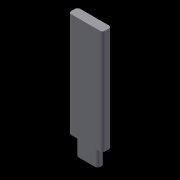
# Autodesk Inventor part: 3d_JacintoDevKit_Addon - USB Type-C
Saved by Autodesk Inventor 2018.3 (Build 223284000, 284)
## iProperties
Created: 2026-02-25
Part Number: 3d_JacintoDevKit_Addon - USB Type-C
Material: Genérico
Document SubType Name: Modeling
Designer: aca6
Density: 1 g/cm^3
Appearance: Valor por defecto
Author: aca6
Autodesk Inventor part; units mm, degrees
ref_plane "YZ Plane" through (0, 0, 0) normal (1, 0, 0) x (0, 1, 0)
ref_plane "XZ Plane" through (0, 0, 0) normal (0, 1, 0) x (-1, 0, 0)
ref_plane "XY Plane" through (0, 0, 0) normal (0, 0, 1) x (1, 0, 0)
sketch "Sketch1" plane through (0, 0, 0) normal (0, 0, 1) x (1, 0, 0)
  line L0 (-5.5, 1.75) -> (5.5, 1.75)
  line L1 (6.5, 0.75) -> (6.5, -0.75)
  line L2 (5.5, -1.75) -> (-5.5, -1.75)
  line L3 (-6.5, -0.75) -> (-6.5, 0.75)
  line L4 (0, 0) -> (0, 3.6789) construction
  line L5 (0, 0) -> (3.0794, 0) construction
  arc A0 (-5.5, 1.75) -> (-6.5, 0.75) centre (-5.5, 0.75) ccw
  arc A1 (-6.5, -0.75) -> (-5.5, -1.75) centre (-5.5, -0.75) ccw
  arc A2 (5.5, -1.75) -> (6.5, -0.75) centre (5.5, -0.75) ccw
  arc A3 (6.5, 0.75) -> (5.5, 1.75) centre (5.5, 0.75) ccw
  point P0 (-6.5, 1.75)
  point P1 (6.5, -1.75)
  point P2 (6.5, 1.75)
  dimension "d0" = 13
  dimension "d1" = 3.5
  dimension "d2" = 1
  dimension "d3" = 1
  constraints: 12 end point, 8 point on circle, 8 tangent, 6 point on line, 4 centre point, 3 horizontal, 2 equal radius, 2 parallel, 2 perpendicular, 1 vertical, 4 other
  measures "d0" distance of point (-6.5, 1.75) point (6.5, 1.75)
  measures "d1" distance of point (6.5, 1.75) point (6.5, -1.75)
  measures "d2" radius of A0
  measures "d3" radius of A1
extrude "Extrusion1" add sketch "Sketch1" along normal blind 40
sketch "Sketch2" plane through (0, 0, 0) normal (0, 0, -1) x (-1, 0, 0)
  line L0 (-3.15, 1.25) -> (3.15, 1.25)
  line L1 (4.15, 0.25) -> (4.15, -0.25)
  line L2 (3.15, -1.25) -> (-3.15, -1.25)
  line L3 (-4.15, -0.25) -> (-4.15, 0.25)
  line L4 (0, 0) -> (0, 2.3167) construction
  line L5 (0, 0) -> (2.0938, 0) construction
  arc A0 (-3.15, 1.25) -> (-4.15, 0.25) centre (-3.15, 0.25) ccw
  arc A1 (-4.15, -0.25) -> (-3.15, -1.25) centre (-3.15, -0.25) ccw
  arc A2 (3.15, -1.25) -> (4.15, -0.25) centre (3.15, -0.25) ccw
  arc A3 (4.15, 0.25) -> (3.15, 1.25) centre (3.15, 0.25) ccw
  point P0 (4.15, -1.25)
  point P1 (4.15, 1.25)
  point P2 (-4.15, -1.25)
  dimension "d6" = 8.3
  dimension "d7" = 2.5
  dimension "d8" = 1
  constraints: 12 end point, 8 point on circle, 8 tangent, 6 point on line, 4 centre point, 3 equal radius, 3 horizontal, 2 parallel, 2 vertical, 1 perpendicular, 4 other
  measures "d6" distance of point (4.15, -1.25) point (-4.15, -1.25)
  measures "d7" distance of point (4.15, 1.25) point (4.15, -1.25)
  measures "d8" radius of A0
extrude "Extrusion2" add sketch "Sketch2" along normal blind 6.5
body "Solid1"
